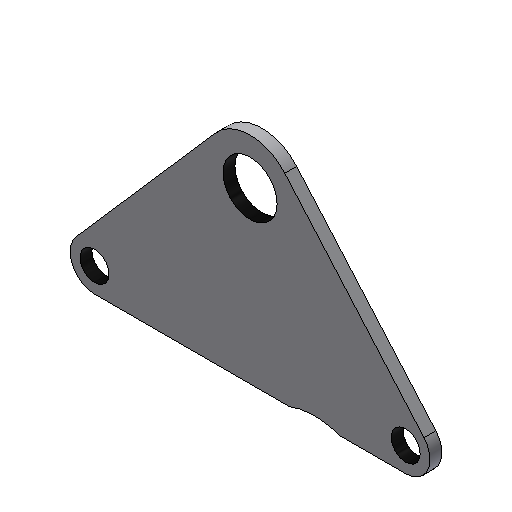
# Autodesk Inventor part: TL20240701-10110CV-021
Saved by Autodesk Inventor 2022.5 (Build 265521000, 521)
## iProperties
Category: DRIVE UNIT ASSY
Manager: 호상태
Company: 현대 트랜시스(대유)
Created: 2023-01-19
Part Number: TL20240701-10110CV-021
Project: SW PJT
Checked By: 김형민
Engr Approved By: 김시현
User Status: 1 x18
Material: SS400
Description: 0
Document SubType Name: Modeling
Mfg Approved By: 호상태
Designer: 박성규
Stock Number: 021
Mass: 1843.21 g
Surface Area: 608.845 cm^2
Volume: 234.804 cm^3
Density: 7.85 g/cm^3
Appearance: Painting-RAL7035
DETAIL: Coveryor Assembly
M/C TITLE: MEa/NEa차종 시트조립라인
SPECIFICATION: TL20221201-000000CV-003
DocNumber: 221118_Standard_v1
Folder: .\
VDS_Category: 엔지니어링
Detail Description: Processed products
Title: TORQUE ARM
Subject: SW차종 시트조립라인
Author: 박성규
Revision Number: A
Autodesk Inventor part; units mm, degrees
ref_plane "YZ Plane" through (0, 0, 0) normal (1, 0, 0) x (0, 1, 0)
ref_plane "XZ Plane" through (0, 0, 0) normal (0, 1, 0) x (-1, 0, 0)
ref_plane "XY Plane" through (0, 0, 0) normal (0, 0, 1) x (1, 0, 0)
sketch "스케치8" plane through (0, 0, 0) normal (0, 0, 1) x (1, 0, 0)
  circle A0 centre (0, 0) radius 35
  circle A1 centre (-118, -110) radius 18.5
  circle A2 centre (118, -110) radius 18.5
  line L0 (-118, -128.5) -> (118, -128.5)
  line L1 (-131.9326, -97.8291) -> (-26.3591, 23.0261)
  line L2 (131.9326, -97.8291) -> (26.3591, 23.0261)
  circle A3 centre (49, -179) radius 54
  point P0 (29.8754, -128.5)
  point P1 (68.1246, -128.5)
  dimension "d38" = 70
  dimension "d39" = 118
  dimension "d40" = 118
  dimension "d41" = 110
  dimension "d42" = 37
  dimension "d43" = 37
  dimension "d60" = 49
  dimension "d61" = 69
  dimension "d62" = 108
  constraints: 6 end point, 6 point on circle, 5 tangent, 4 centre point, 1 coincident, 1 horizontal, 1 horizontal alignment
  measures "d38" diameter of A0
  measures "d39" horizontal distance of point (0, 0) A1.centre
  measures "d40" horizontal distance of A2.centre point (0, 0)
  measures "d41" vertical distance of point (0, 0) A1.centre
  measures "d42" diameter of A1
  measures "d43" diameter of A2
  measures "d60" horizontal distance of A3.centre point (0, 0)
  measures "d61" horizontal distance of A3.centre A2.centre
  measures "d62" diameter of A3
extrude "돌출3" add sketch "스케치8" along normal blind 9 contours A0 | A0 L2 A2 L0 A3 A1 L1 | A2 | A1
sketch "스케치9" plane through (0, 0, 9) normal (0, 0, 1) x (1, 0, 0)
  arc A0 (-131.9326, -97.8291) -> (-118, -128.5) centre (-118, -110) ccw construction
  arc A1 (118, -128.5) -> (131.9326, -97.8291) centre (118, -110) ccw construction
  point P0 (0, 0)
  constraints: 2 coincident
hole "구멍3" at (-118, -110, 9) at (118, -110, 9) direction (0, 0, -1) diameter 22 end through all
sketch "스케치10" plane through (0, 0, 9) normal (0, 0, 1) x (1, 0, 0)
  arc A0 (26.3591, 23.0261) -> (-26.3591, 23.0261) centre (0, 0) ccw construction
  constraints: 1 coincident
hole "구멍4" at (0, 0, 9) direction (0, 0, -1) diameter 41 end through all
equation "\"d43\" = d42"
